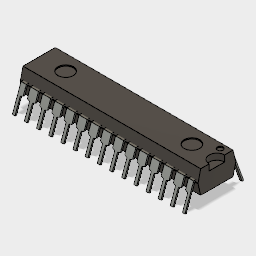
atmega328p v3 (Autodesk Fusion 360 design; units mm, degrees)
Autodesk Fusion 360 part; units mm, degrees
note: some values were not read from the file. Set by a fixed rule: which sketch regions a step uses.
sketch "IC" plane through (0, 0, 0) normal (0, 1, 0) x (1, 0, 0)
  line L0 (0, 0) -> (34.5, 0)
  line L1 (34.5, 0) -> (34.5, -7.3)
  line L2 (34.5, -7.3) -> (0, -7.3)
  line L3 (0, -7.3) -> (0, 0)
  dimension "d1" = 34.5
  dimension "d2" = 7.3
  measures "d1" distance of L0.start L0.end
  measures "d2" distance of L0.start L2.end
extrude "Extrude1" add sketch "IC" along normal blind 4.5 makes body 1
sketch "SideCut" plane through (34.5, 0, 0) normal (1, 0, 0) x (0, 0, -1)
  line L0 (-7.3, 0) -> (0, 0)
  line L1 (0, 0) -> (0, 4.5)
  line L2 (0, 4.5) -> (-7.3, 4.5)
  line L3 (-7.3, 4.5) -> (-7.3, 0)
  line L4 (-7.3, 2.25) -> (0, 2.25) construction
  line L5 (0, 2.2) -> (-7.3, 2.2) construction
  line L6 (-7.3, 2.2) -> (-7.3, 2.3) construction
  line L7 (-7.3, 2.3) -> (0, 2.3) construction
  line L8 (0, 2.3) -> (0, 2.2) construction
  line L9 (0, 2.2) -> (-7.3, 2.3) construction
  line L10 (-7.3, 2.2) -> (0, 2.3) construction
  line L11 (-7.3, 2.2) -> (-6.8, 0)
  line L12 (-7.3, 0) -> (-7.3, 2.2)
  line L13 (-7.3, 0) -> (-6.8, 0)
  line L14 (-3.65, 2.25) -> (-3.65, 6) construction
  line L15 (0, 0) -> (0, 2.2)
  line L16 (0, 2.2) -> (-0.5, 0)
  line L17 (0, 0) -> (-0.5, 0)
  line L18 (0, 2.3) -> (-0.5, 4.5)
  line L19 (0, 4.5) -> (0, 2.3)
  line L20 (0, 4.5) -> (-0.5, 4.5)
  line L21 (-7.3, 2.3) -> (-6.8, 4.5)
  line L22 (-7.3, 4.5) -> (-7.3, 2.3)
  line L23 (-7.3, 4.5) -> (-6.8, 4.5)
  point P0 (-3.65, 2.25)
  dimension "d5" = 0.1
  dimension "d6" = 0.5
  measures "d5" distance of L5 L7
  measures "d6" distance of L11.end L0.start
extrude "Extrude2" cut sketch "SideCut" against normal up to surface (34.5 mm away) contours L0 L3 L11 L12 L13 | L0 L1 L15 L16 L17 | L2 L3 L21 L22 L23 | L1 L2 L18 L19 L20 bodies 1
sketch "TopHoleSide" plane through (0, 4.5, 0) normal (0, 1, 0) x (-1, 0, 0)
  line L0 (0, 6.8) -> (-34.5, 6.8)
  line L1 (-34.5, 6.8) -> (-34.5, 0.5)
  line L2 (-34.5, 0.5) -> (0, 0.5)
  line L3 (0, 0.5) -> (0, 6.8)
  line L4 (0, 3.65) -> (-34.5, 3.65) construction
  circle A0 centre (-34.5, 3.65) radius 1.5
  dimension "d9" = 3
  measures "d9" diameter of A0
extrude "Extrude3" cut sketch "TopHoleSide" against normal blind 1.2 contours L1 A0 picked at (-34.15, 4.1048) bodies 1
sketch "TopHoles" plane through (0, 4.5, 0) normal (0, 1, 0) x (-1, 0, 0)
  arc A0 (-34.5, 2.15) -> (-34.5, 5.15) centre (-34.5, 3.65) ccw
  line L0 (-34.5, 2.15) -> (-34.5, 0.5)
  line L1 (-34.5, 0.5) -> (0, 0.5)
  line L2 (0, 0.5) -> (0, 6.8)
  line L3 (0, 6.8) -> (-34.5, 6.8)
  line L4 (-34.5, 6.8) -> (-34.5, 5.15)
  line L5 (-34.5, 2.15) -> (-34.5, 5.15)
  line L6 (0, 3.5) -> (-34.5, 3.5) construction
  circle A1 centre (-29.5, 3.5) radius 1.5
  circle A2 centre (-5, 3.5) radius 1.5
  circle A3 centre (-33, 1.5) radius 0.55
  dimension "d12" = 5
  dimension "d13" = 5
  dimension "d14" = 1.1
  dimension "d15" = 2
  dimension "d16" = 1.5
  measures "d12" distance of L6.start A2.centre
  measures "d13" distance of L6.end A1.centre
  measures "d14" diameter of A3
  measures "d15" distance of L6.end A3.centre
  measures "d16" distance of L6.end A3.centre
extrude "Extrude4" cut sketch "TopHoles" against normal blind 0.2 contours A1 | A2 | A3 bodies 1
ref_plane "WorkPlane1" through (34, 2.25, 3.65) normal (1, 0, 0) x (0, 0, -1)
copy_body "Body->Comp1" bodies 1 removing the originals makes body 2 in component "IC"
sketch "PinBase" plane through (34, 2.25, 3.65) normal (1, 0, 0) x (0, 0, -1)
  line L0 (3.65, -0.05) -> (3.65, 0.05)
  line L1 (-3.65, 0.05) -> (3.65, 0.05) construction
  line L2 (-3.7899, 0.05) -> (3.7899, 0.05)
  line L3 (3.7899, 0.05) -> (5.4282, -4.4511)
  line L4 (5.4282, -4.4511) -> (5.7101, -4.3485)
  line L5 (5.7101, -4.3485) -> (4, 0.35)
  line L6 (4, 0.35) -> (-4, 0.35)
  line L7 (-4, 0.35) -> (-5.7101, -4.3485)
  line L8 (-5.7101, -4.3485) -> (-5.4282, -4.4511)
  line L9 (-5.4282, -4.4511) -> (-3.7899, 0.05)
  line L10 (0, 1.2) -> (0, -0.7) construction
  point P0 (-3.65, 0.05)
  point P1 (3.65, 0.05)
  dimension "d20" = 8
  dimension "d21" = 0.3
  dimension "d22" = 0.3
  dimension "d23" = 0.3
  dimension "d26" = 110
  dimension "d27" = 110
  dimension "d28" = 4
  dimension "d34" = 5
  dimension "d35" = 5
  measures "d20" distance of L5.end L6.end
  measures "d21" distance of L2 L6
  measures "d22" distance of L7 L9
  measures "d23" distance of L3 L5
  measures "d26" angle of L2 L3
  measures "d27" angle of L2 L9
  measures "d28" distance of L5.end L10
  measures "d34" distance of L6.end L7.end
  measures "d35" distance of L4.end L5.end
extrude "Extrude5" add sketch "PinBase" against normal blind 33.5 separate body makes body 3
ref_plane "WorkPlane2" through (17.25, 2.25, 3.65) normal (0, 0, 1) x (1, 0, 0)
sketch "pinCut" plane through (0, 2.7628, 7.5907) normal (0, 0.34202, 0.939693) x (1, 0, 0)
  line L0 (34, -5.1733) -> (34, -0.1733)
  line L1 (34, -0.1733) -> (0.5, -0.1733)
  line L2 (0.5, -0.1733) -> (0.5, -5.1733)
  line L3 (0.5, -5.1733) -> (34, -5.1733)
  line L4 (34, -1.9733) -> (0.5, -1.9733) construction
  line L5 (34, -5.1733) -> (33, -5.1733) construction
  line L6 (33.5, -5.1733) -> (33.5, -2.1733)
  line L7 (33.5, -2.1733) -> (33, -1.9733)
  line L8 (0, -0.171) -> (34.5, -0.171) construction
  line L9 (33, 1.2567) -> (33, -1.9733)
  line L10 (34, -5.1733) -> (33.75, -5.1733) construction
  line L11 (33.75, -5.1733) -> (31.21, -5.1733) construction
  line L12 (31.21, -5.1733) -> (31.71, -5.1733) construction
  line L13 (33.5, -5.1733) -> (31.71, -5.1733)
  line L14 (31.71, -5.1733) -> (31.71, -2.1733)
  line L15 (31.71, -2.1733) -> (32.21, -1.9733)
  line L16 (32.21, -1.9733) -> (32.21, 1.2567)
  line L17 (32.21, 1.2567) -> (33, 1.2567)
  dimension "d33" = 3.2
  dimension "d36" = 1
  dimension "d37" = 1
  dimension "d38" = 0.2
  dimension "d39" = 0.25
  dimension "d40" = 2.54
  dimension "d41" = 2.54
  dimension "d42" = 0.5
  dimension "d43" = 0.2
  dimension "d44" = 1
  dimension "d47" = 1.43
  measures "d33" distance of L3 L4
  measures "d36" distance of L0.start L5.end
  measures "d37" distance of L0 L9
  measures "d38" distance of L4 L6.end
  measures "d39" distance of L0.start L10.end
  measures "d40" distance of L10.end L11.end
  measures "d41" distance of L10.end L11.end
  measures "d42" distance of L11.end L12.end
  measures "d43" distance of L14.end L15.end
  measures "d44" distance of L11.end L16.end
  measures "d47" distance of L1 L17
extrude "Extrude8" cut sketch "pinCut" against normal blind 2.8 contours L1 L3 L6 L7 L9 L13 L14 L15 L16 | L1 L9 L16 L17 bodies 3
pattern_linear "R-Pattern1" count 14 spacing 2.36 along (-1, 0, 0) of "Extrude8"
mirror "Mirror1" about plane through (17.25, 2.25, 3.65) normal (0, 0, 1) of "Extrude8", "R-Pattern1"
component "IC" placed x (1, 0, 0) y (0, 1, 0) z (0, 0, 1) at (0, 0, 0)
equation "d22 = d21"
equation "d23 = d21"
equation "d27 = d26"
equation "d28 = d20 / 2"
equation "d35 = d34"
equation "d37 = d36"
equation "d43 = d38"
